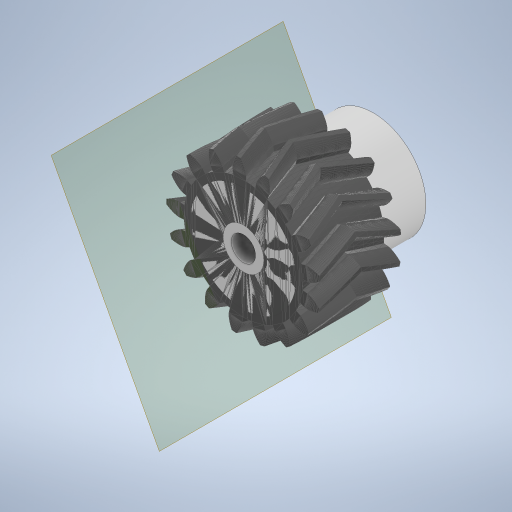
# Autodesk Inventor part: gears_3mm_17TModded
Saved by Autodesk Inventor 2024.2 (Build 282272000, 272)
## iProperties
Created: 2024-06-02
Part Number: gears_3mm_17TModded
Material: Generic
Document SubType Name: Modeling
Designer: Robin
Density: 1 g/cm^3
Appearance: Default
Author: Robin
Autodesk Inventor part; units mm, degrees
ref_plane "YZ Plane" through (0, 0, 0) normal (1, 0, 0) x (0, 1, 0)
ref_plane "XZ Plane" through (0, 0, 0) normal (0, 1, 0) x (-1, 0, 0)
ref_plane "XY Plane" through (0, 0, 0) normal (0, 0, 1) x (1, 0, 0)
sketch "Sketch1" plane through (0.3113, 7.3239, 0) normal (0, 0, -1) x (-1, 0, 0)
  circle A0 centre (0.3113, -7.3239) radius 6.5
  circle A1 centre (0.3113, -7.3239) radius 1.5
  dimension "d0" = 13
  dimension "d1" = 3
  constraints: 2 centre point, 2 coincident
  measures "d0" diameter of A0
  measures "d1" diameter of A1
extrude "Extrusion1" add sketch "Sketch1" along normal blind 6 and the other way blind 10
ref_plane "Work Plane1" through (-5.7325, -3.064, 0) normal (-0.8819, -0.4714, 0) x (0.4714, -0.8819, 0)
sketch "Sketch2" plane through (-5.7325, -3.064, 0) normal (-0.8819, -0.4714, 0) x (0.4714, -0.8819, 0)
  circle A0 centre (0, -2) radius 2
  point P0 (0, 0)
  dimension "d6" = 4
  dimension "d7" = 2
  constraints: 1 centre point
  measures "d6" diameter of A0
  measures "d7" distance of A0.centre point (0, 0)
extrude "Extrusion2" cut sketch "Sketch2" against normal blind 8
body "Solid1"
